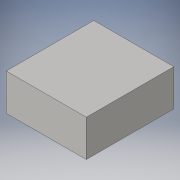
# Autodesk Inventor part: CombinerBlock
Saved by Autodesk Inventor 2016 (Build 200138000, 138)
## iProperties
Created: 2016-08-31
Part Number: CombinerBlock
Material: Generic
Document SubType Name: Modeling
Designer: jfixelle
Density: 1 g/cm^3
Appearance: Default
Author: jfixelle
Autodesk Inventor part; units mm, degrees
ref_plane "YZ Plane" through (0, 0, 0) normal (1, 0, 0) x (0, 1, 0)
ref_plane "XZ Plane" through (0, 0, 0) normal (0, 1, 0) x (-1, 0, 0)
ref_plane "XY Plane" through (0, 0, 0) normal (0, 0, 1) x (1, 0, 0)
sketch "Sketch1" plane through (0, 0, 0) normal (0, 1, 0) x (-1, 0, 0)
  line L0 (10.0765, 11.6952) -> (-11.7675, 11.6952)
  line L1 (-11.7675, 11.6952) -> (-11.7675, -12.1808)
  line L2 (-11.7675, -12.1808) -> (10.0765, -12.1808)
  line L3 (10.0765, -12.1808) -> (10.0765, 11.6952)
  point P0 (0, 0)
  dimension "d0" = 23.876
  dimension "d1" = 21.844
  constraints: 8 end point, 2 parallel, 1 horizontal, 1 perpendicular
  measures "d0" distance of L2.end L0.start
  measures "d1" distance of L1.end L2.end
extrude "Extrusion1" add sketch "Sketch1" along normal blind 10
body "Solid1"
